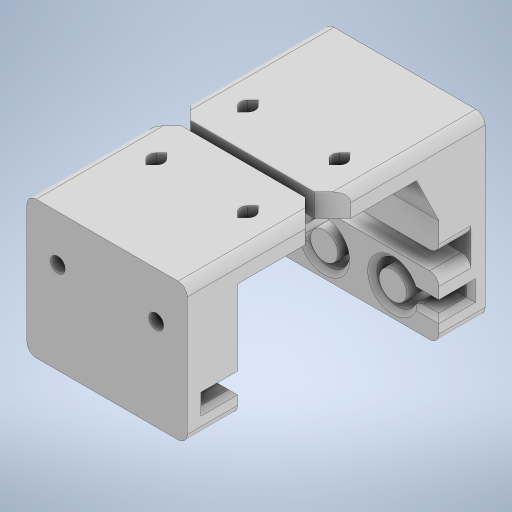
# Autodesk Inventor part: carriage
Saved by Autodesk Inventor 2023.1 (Build 271208000, 208)
## iProperties
Created: 2022-11-02
Part Number: carriage
Material: Generic
Document SubType Name: Modeling
Designer: nicol
Density: 1 g/cm^3
Appearance: Default
Author: nicol
Autodesk Inventor part; units mm, degrees
ref_plane "YZ Plane" through (0, 0, 0) normal (1, 0, 0) x (0, 1, 0)
ref_plane "XZ Plane" through (0, 0, 0) normal (0, 1, 0) x (-1, 0, 0)
ref_plane "XY Plane" through (0, 0, 0) normal (0, 0, 1) x (1, 0, 0)
sketch "Sketch1" plane through (0, 0, 0) normal (0, 1, 0) x (-1, 0, 0)
  line L0 (0, 0) -> (35, 0)
  line L1 (35, 0) -> (35, -65.05)
  line L2 (35, -65.05) -> (0, -65.05)
  line L3 (0, -65.05) -> (0, 0)
  line L4 (27.5, -20.75) -> (7.5, -20.75) construction
  line L5 (7.5, -20.75) -> (7.5, -40.75) construction
  line L6 (7.5, -40.75) -> (27.5, -40.75) construction
  line L7 (27.5, -40.75) -> (27.5, -20.75) construction
  dimension "d0" = 20
  dimension "d1" = 20
  dimension "d2" = 20.75
  dimension "d3" = 24.3
  dimension "d4" = 35
  dimension "d5" = 7.5
  dimension "d6" = 7.5
  constraints: 16 end point, 4 parallel, 2 horizontal, 2 perpendicular
  measures "d0" distance of L6.end L5.end
  measures "d1" distance of L5.end L4.end
  measures "d2" distance between parallel lines of L0 L4
  measures "d3" distance between parallel lines of L2 L6
  measures "d4" distance of L0.start L0.end
  measures "d5" distance between parallel lines of L1 L7
  measures "d6" distance between parallel lines of L3 L5
extrude "Extrusion1" add sketch "Sketch1" against normal blind 5
hole "Hole1" at (-27.5, 0, -20.75) at (-7.5, 0, -20.75) at (-27.5, 0, -40.75) at (-7.5, 0, -40.75) direction (0, -1, 0) diameter 3.2 end through all
sketch "Sketch2" plane through (0, -5, 0) normal (0, -1, 0) x (1, 0, 0)
  circle A0 centre (-27.5, -40.75) radius 1.6 projected
  circle A1 centre (-27.5, -20.75) radius 1.6 projected
  circle A2 centre (-7.5, -20.75) radius 1.6 projected
  circle A3 centre (-7.5, -40.75) radius 1.6 projected
  line L0 (-35, -65.05) -> (0, -65.05) projected
  line L1 (0, -65.05) -> (0, 0) projected
  line L2 (0, 0) -> (-35, 0) projected
  line L3 (-35, 0) -> (-35, -65.05) projected
  line L4 (0, -50.05) -> (-35, -50.05)
  line L5 (-35, -65.05) -> (-35, 0) projected
  line L6 (-35, -11) -> (0, -11)
  line L7 (0, 0) -> (0, -65.05) projected
  point P0 (0, -11)
  dimension "d16" = 11
  dimension "d17" = 15
  constraints: 4 end point, 4 point on line, 1 horizontal, 1 parallel
  measures "d16" distance between parallel lines of L2 L6
  measures "d17" distance between parallel lines of L0 L4
extrude "Extrusion2" add sketch "Sketch2" along normal blind 33.5 contours L3 L4 L1 L0
extrude "Extrusion24" add sketch "Sketch2" along normal blind 25 contours L3 L2 L1 L6
sketch "Sketch26" plane through (-35, 0, -11) normal (0, 0, 1) x (1, 0, 0)
  circle A0 centre (12, -23.75) radius 4.5
  circle A1 centre (12, -23.75) radius 3
  circle A2 centre (23, -23.75) radius 4.5
  circle A3 centre (23, -23.75) radius 3
  line L0 (0, -22.5) -> (12, -22.5)
  line L1 (12, -22.5) -> (12, -25)
  line L2 (12, -25) -> (0, -25)
  line L3 (0, -25) -> (0, -22.5)
  line L4 (35, -22.5) -> (23, -22.5)
  line L5 (23, -22.5) -> (23, -25)
  line L6 (23, -25) -> (35, -25)
  line L7 (35, -25) -> (35, -22.5)
  line L8 (0, 0) -> (0, -30) projected
  line L9 (35, 0) -> (35, -30) projected
  line L10 (25.9, 0) -> (29.1, 0) projected
  line L11 (9.1, -5) -> (5.9, -5) projected
  line L12 (9.1, -5) -> (5.9, -5) projected
  line L13 (29.1, -5) -> (25.9, -5) projected
  line L14 (29.1, -5) -> (25.9, -5) projected
  line L15 (35, -5) -> (0, -5) projected
  line L16 (0, -5) -> (35, -5) projected
  point P0 (27.3229, -22.5)
  point P1 (27.3229, -25)
  point P2 (7.6771, -22.5)
  point P3 (7.6771, -25)
  dimension "d264" = 2.5
  dimension "d265" = 20
  dimension "d266" = 6
  dimension "d267" = 9
  dimension "d268" = 12
  constraints: 16 end point, 5 collinear, 4 centre point, 4 coincident, 4 parallel, 2 equal radius, 2 horizontal, 2 midpoint, 2 perpendicular
  measures "d264" distance between parallel lines of L2 L0
  measures "d265" distance between parallel lines of L2 L15
  measures "d266" diameter of A1
  measures "d267" diameter of A0
  measures "d268" distance of L0.start L0.end
extrude "Extrusion25" cut sketch "Sketch26" along normal blind 7 contours A0 L2 A1 L0 | L0 A1 L2 A0 | A0 L2 L3 L0 | A2 L6 A3 L4 | A2 L4 L7 L6 | L4 A3 L6 A2
chamfer "Chamfer7" distance 1 angle 45 12 edges at (-3.8385, -22.5, -11) (-16.5, -23.75, -11) (-3.8385, -25, -11) (-18.5, -23.75, -11) (-31.1615, -22.5, -11) (-31.1615, -25, -11) (0, -22.5, -7.5) (0, -25, -7.5) (-35, -22.5, -7.5) (-35, -25, -7.5) (0, -23.75, -4) (-35, -23.75, -4)
fillet "Fillet5" radius 2 4 edges at (-7.6771, -22.5, -7) (-7.6771, -25, -7) (-27.3229, -22.5, -7) (-27.3229, -25, -7)
sketch "Sketch27" plane through (-35, -5, -50.05) normal (0, 0, 1) x (1, 0, 0)
  line L0 (0, 0) -> (35, 0) projected
  line L1 (0, 0) -> (0, -33.5) projected
  line L2 (35, -33.5) -> (0, -33.5) projected
  line L3 (35, 0) -> (35, -33.5) projected
  line L4 (0, 0) -> (0, -33.5) projected
  line L5 (0, -10) -> (35, -10)
  line L6 (35, -10) -> (35, -33.5)
  line L7 (35, -33.5) -> (0, -33.5)
  line L8 (0, -33.5) -> (0, -10)
  point P0 (35, 5)
  dimension "d288" = 10
  constraints: 8 end point, 2 parallel, 1 horizontal, 1 perpendicular, 1 point on line
  measures "d288" distance between parallel lines of L0 L5
extrude "Extrusion26" cut sketch "Sketch27" against normal blind 4.9 contours L5 L3 L2 L1
sketch "Sketch25" plane through (-35, -15, -54.95) normal (0, 0, 1) x (1, 0, 0)
  circle A0 centre (25, -17.25) radius 1.6
  circle A1 centre (10, -17.25) radius 1.6
  circle A2 centre (25, -17.25) radius 3
  circle A3 centre (10, -17.25) radius 3
  line L0 (25, -16) -> (35, -16)
  line L1 (35, -16) -> (35, -18.5)
  line L2 (35, -18.5) -> (25, -18.5)
  line L3 (25, -18.5) -> (25, -16) construction
  line L4 (10, -16) -> (0, -16)
  line L5 (0, -16) -> (0, -18.5)
  line L6 (0, -18.5) -> (10, -18.5)
  line L7 (10, -18.5) -> (10, -16)
  line L8 (0, -23.5) -> (35, -23.5)
  circle A4 centre (25, -17.25) radius 4.5
  line L9 (0, -6.5) -> (35, -6.5)
  line L10 (35, -6.5) -> (35, -10.5)
  line L11 (35, -10.5) -> (0, -10.5)
  line L12 (0, -10.5) -> (0, -6.5)
  circle A5 centre (10, -17.25) radius 4.5
  line L13 (0, -23.5) -> (0, 0) projected
  line L14 (35, -23.5) -> (0, -23.5) projected
  line L15 (35, 0) -> (35, -23.5) projected
  line L16 (0, 0) -> (35, 0) projected
  line L17 (35, -23.5) -> (0, -23.5) projected
  line L18 (0, -23.5) -> (0, 0) projected
  line L19 (35, 0) -> (35, -23.5) projected
  point P0 (35, 15)
  point P1 (29.3229, -16)
  point P2 (29.3229, -18.5)
  point P3 (5.6771, -18.5)
  point P4 (5.6771, -16)
  dimension "d240" = 5
  dimension "d241" = 2.5
  dimension "d242" = 3.2
  dimension "d243" = 6
  dimension "d244" = 9
  dimension "d245" = 4
  dimension "d247" = 17
  dimension "d248" = 10
  constraints: 26 end point, 8 collinear, 6 centre point, 6 coincident, 6 parallel, 3 equal radius, 3 horizontal, 3 perpendicular, 2 midpoint
  measures "d240" distance between parallel lines of L8 L2
  measures "d241" distance of L0.end L1.end
  measures "d242" diameter of A0
  measures "d243" diameter of A2
  measures "d244" diameter of A4
  measures "d245" distance of L9.end L10.end
  measures "d247" distance between parallel lines of L8 L9
  measures "d248" distance of L0.start L0.end
extrude "Extrusion23" cut sketch "Sketch25" against normal blind 7 contours L0 A4 L2 A2 | A2 L2 A4 L0 | L0 L1 L2 A4 | L11 L12 L9 L10 | L4 A5 L6 L5 | A5 L6 A3 L4 | L4 A3 L6 A5
chamfer "Chamfer6" distance 1 angle 45 12 edges at (-35, -32.25, -61.95) (0, -32.25, -61.95) (-35, -31, -58.45) (-35, -33.5, -58.45) (-32.1615, -31, -54.95) (-32.1615, -33.5, -54.95) (-20.5, -32.25, -54.95) (-14.5, -32.25, -54.95) (-2.8385, -31, -54.95) (-2.8385, -33.5, -54.95) (0, -33.5, -58.45) (0, -31, -58.45)
fillet "Fillet4" radius 2 4 edges at (-5.6771, -31, -58.95) (-5.6771, -33.5, -58.95) (-29.3229, -33.5, -58.95) (-29.3229, -31, -58.95)
sketch "Sketch14" plane through (-35, -25, 0) normal (0, 0, 1) x (1, 0, 0)
  line L0 (9.55, 13.3834) -> (6.75, 11.7668)
  line L1 (6.75, 11.7668) -> (3.95, 13.3834)
  line L2 (3.95, 13.3834) -> (3.95, 16.6166)
  line L3 (3.95, 16.6166) -> (6.75, 18.2332)
  line L4 (6.75, 18.2332) -> (9.55, 16.6166)
  line L5 (9.55, 16.6166) -> (9.55, 13.3834)
  line L6 (28.25, 11.7668) -> (25.45, 13.3834)
  line L7 (25.45, 13.3834) -> (25.45, 16.6166)
  line L8 (25.45, 16.6166) -> (28.25, 18.2332)
  line L9 (28.25, 18.2332) -> (31.05, 16.6166)
  line L10 (31.05, 16.6166) -> (31.05, 13.3834)
  line L11 (31.05, 13.3834) -> (28.25, 11.7668)
  line L12 (0, 25) -> (35, 25) projected
  line L13 (0, 25) -> (0, -5) projected
  line L14 (35, 25) -> (35, -5) projected
  point P0 (6.75, 15)
  point P1 (28.25, 15)
  point P2 (0, 2.5)
  point P3 (35, 2.5)
  dimension "d120" = 5.6
  dimension "d271" = 21.5
  dimension "d274" = 10
  dimension "d275" = 6.75
  dimension "d276" = 6.75
  constraints: 24 end point, 2 vertical, 1 horizontal alignment, 1 parallel, 26 other
  measures "d120" distance between parallel lines of L5 L2
  measures "d271" distance of point (28.25, 15) point (6.75, 15)
  measures "d274" distance from line of L12 point (6.75, 15)
  measures "d275" distance from line of point (6.75, 15) L13
  measures "d276" distance from line of L14 point (28.25, 15)
extrude "Extrusion12" cut sketch "Sketch14" along normal blind 8 from surface at -11
hole "Hole4" at (-6.75, -10, 0) at (-28.25, -10, 0) direction (0, 0, -1) diameter 3.2 depth 11 tip angle 118
sketch "Sketch22" plane through (0, 0, 0) normal (0, 1, 0) x (1, 0, 0)
  line L0 (16.0256, 29.75) -> (-78.6573, 29.75)
  line L1 (-78.6573, 29.75) -> (-78.6573, 31.75)
  line L2 (-78.6573, 31.75) -> (16.0256, 31.75)
  line L3 (16.0256, 31.75) -> (16.0256, 29.75)
  circle A0 centre (-7.5, 20.75) radius 1.6 projected
  circle A1 centre (-7.5, 40.75) radius 1.6 projected
  line L4 (-7.5, 20.75) -> (-7.5, 40.75) construction
  point P0 (0, 0)
  point P1 (-31.3158, 29.75)
  point P2 (-7.5, 30.75)
  point P3 (16.0256, 30.75)
  dimension "d195" = 2
  constraints: 10 end point, 3 midpoint, 2 parallel, 1 horizontal, 1 horizontal alignment, 1 perpendicular, 1 vertical
  measures "d195" distance from line of point (-31.316, 29.75) L2
extrude "Extrusion20" cut sketch "Sketch22" against normal through all contours L0 L1 L2 L3
chamfer "Chamfer3" distance 4 angle 45 4 edges at (0, -2.5, -29.75) (0, -2.5, -31.75) (-35, -2.5, -29.75) (-35, -2.5, -31.75)
chamfer "Chamfer4" distance 10 distance2 4.9 1 edges at (-17.5, -15, -50.05) measured on face at (-17.5, -14.5, -50.05)
fillet "Fillet3" radius 2 12 edges at (0, 0, -50.4) (-35, 0, -50.4) (-35, 0, -12.875) (0, 0, -12.875) (0, -30, -5.5) (-35, -30, -5.5) (-35, -21.5, -58.45) (-35, -25.5, -58.45) (0, -21.5, -58.45) (0, -25.5, -58.45) (-35, -38.5, -60) (0, -38.5, -60)
sketch "Sketch24" plane through (0, 0, 0) normal (0, 1, 0) x (1, 0, 0)
  circle A0 centre (-27.5, 40.75) radius 1.6 projected
  circle A1 centre (-7.5, 40.75) radius 1.6 projected
  line L0 (-7.5, 43.0127) -> (-9.7627, 40.75)
  line L1 (-9.7627, 40.75) -> (-7.5, 38.4873)
  line L2 (-7.5, 38.4873) -> (-5.2373, 40.75)
  line L3 (-5.2373, 40.75) -> (-7.5, 43.0127)
  circle A2 centre (-7.5, 40.75) radius 1.6 projected
  line L4 (-7.5, 43.0127) -> (-7.5, 38.4873) construction
  line L5 (-9.7627, 40.75) -> (-5.2373, 40.75) construction
  line L6 (-7.5, 43.0127) -> (-4.3, 43.0127) construction
  line L7 (-27.5, 43.0127) -> (-29.7627, 40.75)
  line L8 (-29.7627, 40.75) -> (-27.5, 38.4873)
  line L9 (-27.5, 38.4873) -> (-25.2373, 40.75)
  line L10 (-25.2373, 40.75) -> (-27.5, 43.0127)
  circle A3 centre (-27.5, 40.75) radius 1.6 projected
  line L11 (-27.5, 43.0127) -> (-27.5, 38.4873) construction
  line L12 (-29.7627, 40.75) -> (-25.2373, 40.75) construction
  line L13 (-27.5, 18.4873) -> (-29.7627, 20.75)
  line L14 (-29.7627, 20.75) -> (-27.5, 23.0127)
  line L15 (-27.5, 23.0127) -> (-25.2373, 20.75)
  line L16 (-25.2373, 20.75) -> (-27.5, 18.4873)
  line L17 (-27.5, 18.4873) -> (-27.5, 23.0127) construction
  line L18 (-29.7627, 20.75) -> (-25.2373, 20.75) construction
  line L19 (-7.5, 18.4873) -> (-9.7627, 20.75)
  line L20 (-9.7627, 20.75) -> (-7.5, 23.0127)
  line L21 (-7.5, 23.0127) -> (-5.2373, 20.75)
  line L22 (-5.2373, 20.75) -> (-7.5, 18.4873)
  circle A4 centre (-7.5, 20.75) radius 1.6 projected
  line L23 (-7.5, 18.4873) -> (-7.5, 23.0127) construction
  line L24 (-9.7627, 20.75) -> (-5.2373, 20.75) construction
  circle A5 centre (-27.5, 20.75) radius 1.6 projected
  point P0 (0, 0)
  point P1 (-6.3686, 39.6186)
  point P2 (-8.6314, 39.6186)
  point P3 (-26.3686, 39.6186)
  point P4 (-28.6314, 39.6186)
  point P5 (-2, 0)
  point P6 (-33, 27.75)
  point P7 (-6.3686, 41.8814)
  point P8 (-8.6314, 41.8814)
  point P9 (-26.3686, 41.8814)
  point P10 (-28.6314, 41.8814)
  point P11 (-6.3686, 21.8814)
  point P12 (-8.6314, 21.8814)
  point P13 (-8.6314, 19.6186)
  point P14 (-6.3686, 19.6186)
  point P15 (-26.3686, 21.8814)
  point P16 (-28.6314, 21.8814)
  point P17 (-28.6314, 19.6186)
  point P18 (-26.3686, 19.6186)
  dimension "d237" = 135
  constraints: 50 end point, 9 parallel, 6 midpoint, 6 tangent, 4 perpendicular, 3 vertical, 2 centre point, 1 equal length, 1 horizontal
  measures "d237" angle of L0 L6
extrude "Extrusion22" cut sketch "Sketch24" against normal blind 10 contours A0 L7 L10 | L9 L8 A0 | A1 L0 L3 | L2 L1 A1 | L13 A5 L16 | A5 | L14 L15 A5 | L19 A4 L22 | A4 | L20 L21 A4
ref_plane "Work Plane5" through (-4, 0, -30.75) normal (0, 0, -1) x (-1, 0, 0)
equation "\"d5\" = d6"
body "Solid1"
